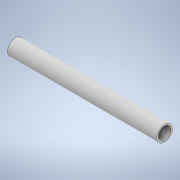
# Autodesk Inventor part: buis
Saved by Autodesk Inventor 2020.1 (Build 241239000, 239)
## iProperties
Created: 2019-11-19
Part Number: buis
Material: Generic
Document SubType Name: Modeling
Designer: jonas.vandenborne
Density: 1 g/cm^3
Appearance: Default
Author: jonas.vandenborne
Autodesk Inventor part; units mm, degrees
ref_plane "YZ Plane" through (0, 0, 0) normal (1, 0, 0) x (0, 1, 0)
ref_plane "XZ Plane" through (0, 0, 0) normal (0, 1, 0) x (-1, 0, 0)
ref_plane "XY Plane" through (0, 0, 0) normal (0, 0, 1) x (1, 0, 0)
sketch "Sketch1" plane through (0, 0, 0) normal (0, 0, 1) x (1, 0, 0)
  line L0 (0, 8.5) -> (200, 8.5)
  line L1 (200, 8.5) -> (200, 10.5)
  line L2 (200, 10.5) -> (0, 10.5)
  line L3 (0, 10.5) -> (0, 8.5)
  line L4 (0, 0) -> (200, 0)
  dimension "d0" = 200
  dimension "d1" = 2
  dimension "d4" = 21
  constraints: 10 end point, 3 perpendicular, 2 horizontal
  measures "d0" distance of L1.end L2.end
  measures "d1" distance of L2.end L0.start
  measures "d4" diameter of L2 L4
revolve "Revolution1" add sketch "Sketch1" angle 360 about axis through (0, 0, 0) along (1, 0, 0)
body "Solid1"
